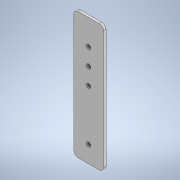
# Autodesk Inventor part: 4
Saved by Autodesk Inventor 2021 (Build 250183000, 183)
## iProperties
Created: 2021-03-30
Part Number: 4
Material: Genérico
Document SubType Name: Modeling
Designer: diego
Density: 1 g/cm^3
Appearance: Valor por defecto
Author: diego
Autodesk Inventor part; units mm, degrees
ref_plane "YZ Plane" through (0, 0, 0) normal (1, 0, 0) x (0, 1, 0)
ref_plane "XZ Plane" through (0, 0, 0) normal (0, 1, 0) x (-1, 0, 0)
ref_plane "XY Plane" through (0, 0, 0) normal (0, 0, 1) x (1, 0, 0)
sketch "Boceto1" plane through (0, 0, 0) normal (0, 0, 1) x (1, 0, 0)
  line L0 (0, 5) -> (0, 145)
  line L1 (5, 150) -> (30, 150)
  line L2 (35, 145) -> (35, 5)
  line L3 (30, 0) -> (5, 0)
  arc A0 (35, 145) -> (30, 150) centre (30, 145) ccw
  arc A1 (5, 150) -> (0, 145) centre (5, 145) ccw
  arc A2 (0, 5) -> (5, 0) centre (5, 5) ccw
  arc A3 (30, 0) -> (35, 5) centre (30, 5) ccw
  circle A4 centre (17.5, 120) radius 2.5
  circle A5 centre (17.5, 100) radius 2.5
  circle A6 centre (17.5, 80) radius 2.5
  circle A7 centre (17.5, 20) radius 2.5
  point P0 (0, 0)
  constraints: 8 centre point, 8 end point, 8 point on circle, 8 tangent, 3 equal radius, 2 perpendicular, 2 point on line, 1 vertical
extrude "Extrusión1" add sketch "Boceto1" along normal blind 3
